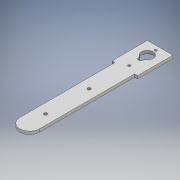
# Autodesk Inventor part: Część2
Saved by Autodesk Inventor 2017 (Build 210142000, 142)
## iProperties
Created: 2017-05-10
Part Number: Część2
Material: Ogólny
Document SubType Name: Modeling
Designer: Damian
Density: 1 g/cm^3
Appearance: Domyślna
Author: Damian
Autodesk Inventor part; units mm, degrees
ref_plane "YZ Plane" through (0, 0, 0) normal (1, 0, 0) x (0, 1, 0)
ref_plane "XZ Plane" through (0, 0, 0) normal (0, 1, 0) x (-1, 0, 0)
ref_plane "XY Plane" through (0, 0, 0) normal (0, 0, 1) x (1, 0, 0)
sketch "Szkic1" plane through (0, 0, 0) normal (0, 0, 1) x (1, 0, 0)
  line L0 (-10, 0) -> (-10, 0)
  line L1 (-20, 10) -> (-20, 107)
  line L2 (0, 107) -> (0, 10)
  arc A0 (-20, 10) -> (-10, 0) centre (-10, 10) ccw
  arc A1 (-10, 0) -> (0, 10) centre (-10, 10) ccw
  line L3 (-23, 143) -> (-23, 107)
  line L4 (3, 107) -> (3, 143)
  line L5 (3, 143) -> (-23, 143)
  line L6 (-23, 143) -> (3, 107) construction
  line L7 (-23, 107) -> (3, 143) construction
  line L8 (-23, 107) -> (-20, 107)
  line L9 (0, 107) -> (3, 107)
  arc A2 (-7.6923, 124.4615) -> (-12.3077, 124.4615) centre (-10, 130) ccw
  arc A3 (-12.3077, 124.4615) -> (-7.6923, 124.4615) centre (-10, 123.5) ccw
  circle A4 centre (-10, 111.5) radius 1.25
  circle A5 centre (-10, 138.5) radius 1.25
  point P0 (0, 0)
  point P1 (-10, 125)
  dimension "d2" = 10
  dimension "d3" = 26
  dimension "d4" = 36
  dimension "d5" = 20
  dimension "d10" = 3
  dimension "d13" = 5
  dimension "d19" = 2.5
  dimension "d20" = 2.5
  dimension "d22" = 6
  dimension "d23" = 13
  dimension "d24" = 13
  dimension "d25" = 6.5
  dimension "d26" = 13
  dimension "d27" = 4.5
  dimension "d28" = 31.5
  dimension "d29" = 13
  dimension "d30" = 120
  dimension "d31" = 36
  constraints: 20 end point, 8 point on circle, 6 centre point, 4 coincident, 4 parallel, 4 perpendicular, 4 tangent, 2 midpoint, 2 point on line, 1 concentric, 1 horizontal
  measures "d2" radius of A0
  measures "d3" distance of L4.start L3.end
  measures "d4" distance of L4.start L4.end
  measures "d5" distance between parallel lines of L2 L1
  measures "d10" distance of L2.start L4.start
  measures "d13" diameter of A3
  measures "d19" diameter of A4
  measures "d20" diameter of A5
  measures "d22" radius of A2
  measures "d23" distance from line of L5 A2.centre
  measures "d24" distance from line of L3 A2.centre
  measures "d25" distance of A2.centre A3.centre
  measures "d26" distance from line of L3 A3.centre
  measures "d27" distance from line of L5 A5.centre
  measures "d28" distance from line of L5 A4.centre
  measures "d29" distance from line of L3 point (-10, 111.5)
  measures "d30" distance of A2.centre A0.centre
  measures "d31" distance of L3.start L3.end
extrude "Wyciągnięcie proste1" add sketch "Szkic1" along normal blind 3
sketch "Szkic2" plane through (0, 0, 3) normal (0, 0, 1) x (1, 0, 0)
  point P0 (0, 0)
  point P1 (-10, 26.1468)
  point P2 (-10, 70.5805)
hole "Otwór1" at (-10, 26.1468, 3) at (-10, 70.5805, 3) direction (0, 0, -1) diameter 3.2 end through all
